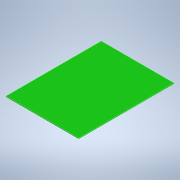
# Autodesk Inventor part: Mock Module PCB
Saved by Autodesk Inventor 2022 (Build 260153000, 153)
## iProperties
Created: 2021-07-19
Part Number: Mock Module PCB
Material: Generic
Document SubType Name: Modeling
Designer: Caleb
Density: 1 g/cm^3
Appearance: Dark Green
Author: Caleb
Autodesk Inventor part; units mm, degrees
(part 1 of 3)
ref_plane "YZ Plane" through (0, 0, 0) normal (1, 0, 0) x (0, 1, 0)
ref_plane "XZ Plane" through (0, 0, 0) normal (0, 1, 0) x (-1, 0, 0)
ref_plane "XY Plane" through (0, 0, 0) normal (0, 0, 1) x (1, 0, 0)
sketch "Sketch1" plane through (0, 0, 0) normal (0, 1, 0) x (-1, 0, 0)
  line L0 (-21.55, 28.25) -> (21.55, 28.25)
  line L1 (21.55, 28.25) -> (21.55, -28.25)
  line L2 (21.55, -28.25) -> (-21.55, -28.25)
  line L3 (-21.55, -28.25) -> (-21.55, 28.25)
  line L4 (-21.55, 28.25) -> (21.55, -28.25) construction
  line L5 (21.55, 28.25) -> (-21.55, -28.25) construction
  point P0 (0, 0)
  dimension "d0" = 43.1
  dimension "d1" = 56.5
  constraints: 12 end point, 2 midpoint, 2 parallel, 1 horizontal, 1 perpendicular
  measures "d0" distance of L0.start L0.end
  measures "d1" distance of L0.end L1.end
extrude "Extrusion1" add sketch "Sketch1" along normal blind 0.5
sketch "Sketch8" plane through (0, 0, 0) normal (0, -1, 0) x (1, 0, 0)
  line L0 (18.3, 26.35) -> (18.2, 26.35)
  line L1 (18.2, 26.35) -> (18.2, 26.05)
  line L2 (18.2, 26.05) -> (18.3, 26.05)
  line L3 (18.3, 26.05) -> (18.3, 26.35)
  line L4 (21.55, 28.25) -> (21.55, -28.25) projected
  line L5 (-21.55, 28.25) -> (21.55, 28.25) projected
  line L6 (18.05, 26.35) -> (17.95, 26.35)
  line L7 (17.95, 26.35) -> (17.95, 26.05)
  line L8 (17.95, 26.05) -> (18.05, 26.05)
  line L9 (18.05, 26.05) -> (18.05, 26.35)
  line L10 (17.8, 26.35) -> (17.7, 26.35)
  line L11 (17.7, 26.35) -> (17.7, 26.05)
  line L12 (17.7, 26.05) -> (17.8, 26.05)
  line L13 (17.8, 26.05) -> (17.8, 26.35)
  line L14 (17.55, 26.35) -> (17.45, 26.35)
  line L15 (17.45, 26.35) -> (17.45, 26.05)
  line L16 (17.45, 26.05) -> (17.55, 26.05)
  line L17 (17.55, 26.05) -> (17.55, 26.35)
  line L18 (17.3, 26.35) -> (17.2, 26.35)
  line L19 (17.2, 26.35) -> (17.2, 26.05)
  line L20 (17.2, 26.05) -> (17.3, 26.05)
  line L21 (17.3, 26.05) -> (17.3, 26.35)
  line L22 (17.05, 26.35) -> (16.95, 26.35)
  line L23 (16.95, 26.35) -> (16.95, 26.05)
  line L24 (16.95, 26.05) -> (17.05, 26.05)
  line L25 (17.05, 26.05) -> (17.05, 26.35)
  line L26 (16.8, 26.35) -> (16.7, 26.35)
  line L27 (16.7, 26.35) -> (16.7, 26.05)
  line L28 (16.7, 26.05) -> (16.8, 26.05)
  line L29 (16.8, 26.05) -> (16.8, 26.35)
  line L30 (16.55, 26.35) -> (16.45, 26.35)
  line L31 (16.45, 26.35) -> (16.45, 26.05)
  line L32 (16.45, 26.05) -> (16.55, 26.05)
  line L33 (16.55, 26.05) -> (16.55, 26.35)
  line L34 (16.3, 26.35) -> (16.2, 26.35)
  line L35 (16.2, 26.35) -> (16.2, 26.05)
  line L36 (16.2, 26.05) -> (16.3, 26.05)
  line L37 (16.3, 26.05) -> (16.3, 26.35)
  line L38 (16.05, 26.35) -> (15.95, 26.35)
  line L39 (15.95, 26.35) -> (15.95, 26.05)
  line L40 (15.95, 26.05) -> (16.05, 26.05)
  line L41 (16.05, 26.05) -> (16.05, 26.35)
  line L42 (15.8, 26.35) -> (15.7, 26.35)
  line L43 (15.7, 26.35) -> (15.7, 26.05)
  line L44 (15.7, 26.05) -> (15.8, 26.05)
  line L45 (15.8, 26.05) -> (15.8, 26.35)
  line L46 (15.55, 26.35) -> (15.45, 26.35)
  line L47 (15.45, 26.35) -> (15.45, 26.05)
  line L48 (15.45, 26.05) -> (15.55, 26.05)
  line L49 (15.55, 26.05) -> (15.55, 26.35)
  line L50 (15.3, 26.35) -> (15.2, 26.35)
  line L51 (15.2, 26.35) -> (15.2, 26.05)
  line L52 (15.2, 26.05) -> (15.3, 26.05)
  line L53 (15.3, 26.05) -> (15.3, 26.35)
  line L54 (15.05, 26.35) -> (14.95, 26.35)
  line L55 (14.95, 26.35) -> (14.95, 26.05)
  line L56 (14.95, 26.05) -> (15.05, 26.05)
  line L57 (15.05, 26.05) -> (15.05, 26.35)
  line L58 (14.8, 26.35) -> (14.7, 26.35)
  line L59 (14.7, 26.35) -> (14.7, 26.05)
  line L60 (14.7, 26.05) -> (14.8, 26.05)
  line L61 (14.8, 26.05) -> (14.8, 26.35)
  line L62 (14.55, 26.35) -> (14.45, 26.35)
  line L63 (14.45, 26.35) -> (14.45, 26.05)
  line L64 (14.45, 26.05) -> (14.55, 26.05)
  line L65 (14.55, 26.05) -> (14.55, 26.35)
  line L66 (14.3, 26.35) -> (14.2, 26.35)
  line L67 (14.2, 26.35) -> (14.2, 26.05)
  line L68 (14.2, 26.05) -> (14.3, 26.05)
  line L69 (14.3, 26.05) -> (14.3, 26.35)
  line L70 (14.05, 26.35) -> (13.95, 26.35)
  line L71 (13.95, 26.35) -> (13.95, 26.05)
  line L72 (13.95, 26.05) -> (14.05, 26.05)
  line L73 (14.05, 26.05) -> (14.05, 26.35)
  line L74 (13.8, 26.35) -> (13.7, 26.35)
  line L75 (13.7, 26.35) -> (13.7, 26.05)
  line L76 (13.7, 26.05) -> (13.8, 26.05)
  line L77 (13.8, 26.05) -> (13.8, 26.35)
  line L78 (13.55, 26.35) -> (13.45, 26.35)
  line L79 (13.45, 26.35) -> (13.45, 26.05)
  line L80 (13.45, 26.05) -> (13.55, 26.05)
  line L81 (13.55, 26.05) -> (13.55, 26.35)
  line L82 (13.3, 26.35) -> (13.2, 26.35)
  line L83 (13.2, 26.35) -> (13.2, 26.05)
  line L84 (13.2, 26.05) -> (13.3, 26.05)
  line L85 (13.3, 26.05) -> (13.3, 26.35)
  line L86 (13.05, 26.35) -> (12.95, 26.35)
  line L87 (12.95, 26.35) -> (12.95, 26.05)
  line L88 (12.95, 26.05) -> (13.05, 26.05)
  line L89 (13.05, 26.05) -> (13.05, 26.35)
  line L90 (12.8, 26.35) -> (12.7, 26.35)
  line L91 (12.7, 26.35) -> (12.7, 26.05)
  line L92 (12.7, 26.05) -> (12.8, 26.05)
  line L93 (12.8, 26.05) -> (12.8, 26.35)
  line L94 (12.55, 26.35) -> (12.45, 26.35)
  line L95 (12.45, 26.35) -> (12.45, 26.05)
  line L96 (12.45, 26.05) -> (12.55, 26.05)
  line L97 (12.55, 26.05) -> (12.55, 26.35)
  line L98 (12.3, 26.35) -> (12.2, 26.35)
  line L99 (12.2, 26.35) -> (12.2, 26.05)
  line L100 (12.2, 26.05) -> (12.3, 26.05)
  line L101 (12.3, 26.05) -> (12.3, 26.35)
  line L102 (12.05, 26.35) -> (11.95, 26.35)
  line L103 (11.95, 26.35) -> (11.95, 26.05)
  line L104 (11.95, 26.05) -> (12.05, 26.05)
  line L105 (12.05, 26.05) -> (12.05, 26.35)
  line L106 (11.8, 26.35) -> (11.7, 26.35)
  line L107 (11.7, 26.35) -> (11.7, 26.05)
  line L108 (11.7, 26.05) -> (11.8, 26.05)
  line L109 (11.8, 26.05) -> (11.8, 26.35)
  line L110 (11.55, 26.35) -> (11.45, 26.35)
  line L111 (11.45, 26.35) -> (11.45, 26.05)
  line L112 (11.45, 26.05) -> (11.55, 26.05)
  line L113 (11.55, 26.05) -> (11.55, 26.35)
  line L114 (11.3, 26.35) -> (11.2, 26.35)
  line L115 (11.2, 26.35) -> (11.2, 26.05)
  line L116 (11.2, 26.05) -> (11.3, 26.05)
  line L117 (11.3, 26.05) -> (11.3, 26.35)
  line L118 (11.05, 26.35) -> (10.95, 26.35)
  line L119 (10.95, 26.35) -> (10.95, 26.05)
  line L120 (10.95, 26.05) -> (11.05, 26.05)
  line L121 (11.05, 26.05) -> (11.05, 26.35)
  line L122 (10.8, 26.35) -> (10.7, 26.35)
  line L123 (10.7, 26.35) -> (10.7, 26.05)
  line L124 (10.7, 26.05) -> (10.8, 26.05)
  line L125 (10.8, 26.05) -> (10.8, 26.35)
  line L126 (10.55, 26.35) -> (10.45, 26.35)
  line L127 (10.45, 26.35) -> (10.45, 26.05)
  line L128 (10.45, 26.05) -> (10.55, 26.05)
  line L129 (10.55, 26.05) -> (10.55, 26.35)
  line L130 (10.3, 26.35) -> (10.2, 26.35)
  line L131 (10.2, 26.35) -> (10.2, 26.05)
  line L132 (10.2, 26.05) -> (10.3, 26.05)
  line L133 (10.3, 26.05) -> (10.3, 26.35)
  line L134 (10.05, 26.35) -> (9.95, 26.35)
  line L135 (9.95, 26.35) -> (9.95, 26.05)
  line L136 (9.95, 26.05) -> (10.05, 26.05)
  line L137 (10.05, 26.05) -> (10.05, 26.35)
  line L138 (9.8, 26.35) -> (9.7, 26.35)
  line L139 (9.7, 26.35) -> (9.7, 26.05)
  line L140 (9.7, 26.05) -> (9.8, 26.05)
  line L141 (9.8, 26.05) -> (9.8, 26.35)
  line L142 (9.55, 26.35) -> (9.45, 26.35)
  line L143 (9.45, 26.35) -> (9.45, 26.05)
  line L144 (9.45, 26.05) -> (9.55, 26.05)
  line L145 (9.55, 26.05) -> (9.55, 26.35)
  line L146 (9.3, 26.35) -> (9.2, 26.35)
  line L147 (9.2, 26.35) -> (9.2, 26.05)
  line L148 (9.2, 26.05) -> (9.3, 26.05)
  line L149 (9.3, 26.05) -> (9.3, 26.35)
  line L150 (9.05, 26.35) -> (8.95, 26.35)
  line L151 (8.95, 26.35) -> (8.95, 26.05)
  line L152 (8.95, 26.05) -> (9.05, 26.05)
  line L153 (9.05, 26.05) -> (9.05, 26.35)
  line L154 (8.8, 26.35) -> (8.7, 26.35)
  line L155 (8.7, 26.35) -> (8.7, 26.05)
  line L156 (8.7, 26.05) -> (8.8, 26.05)
  line L157 (8.8, 26.05) -> (8.8, 26.35)
  line L158 (8.55, 26.35) -> (8.45, 26.35)
  line L159 (8.45, 26.35) -> (8.45, 26.05)
  line L160 (8.45, 26.05) -> (8.55, 26.05)
  line L161 (8.55, 26.05) -> (8.55, 26.35)
  line L162 (8.3, 26.35) -> (8.2, 26.35)
  line L163 (8.2, 26.35) -> (8.2, 26.05)
  line L164 (8.2, 26.05) -> (8.3, 26.05)
  line L165 (8.3, 26.05) -> (8.3, 26.35)
  line L166 (8.05, 26.35) -> (7.95, 26.35)
  line L167 (7.95, 26.35) -> (7.95, 26.05)
  line L168 (7.95, 26.05) -> (8.05, 26.05)
  line L169 (8.05, 26.05) -> (8.05, 26.35)
  line L170 (7.8, 26.35) -> (7.7, 26.35)
  line L171 (7.7, 26.35) -> (7.7, 26.05)
  line L172 (7.7, 26.05) -> (7.8, 26.05)
  line L173 (7.8, 26.05) -> (7.8, 26.35)
  line L174 (7.55, 26.35) -> (7.45, 26.35)
  line L175 (7.45, 26.35) -> (7.45, 26.05)
  line L176 (7.45, 26.05) -> (7.55, 26.05)
  line L177 (7.55, 26.05) -> (7.55, 26.35)
  line L178 (7.3, 26.35) -> (7.2, 26.35)
  line L179 (7.2, 26.35) -> (7.2, 26.05)
  line L180 (7.2, 26.05) -> (7.3, 26.05)
  line L181 (7.3, 26.05) -> (7.3, 26.35)
  line L182 (7.05, 26.35) -> (6.95, 26.35)
  line L183 (6.95, 26.35) -> (6.95, 26.05)
  line L184 (6.95, 26.05) -> (7.05, 26.05)
  line L185 (7.05, 26.05) -> (7.05, 26.35)
  line L186 (6.8, 26.35) -> (6.7, 26.35)
  line L187 (6.7, 26.35) -> (6.7, 26.05)
  line L188 (6.7, 26.05) -> (6.8, 26.05)
  line L189 (6.8, 26.05) -> (6.8, 26.35)
  line L190 (6.55, 26.35) -> (6.45, 26.35)
  line L191 (6.45, 26.35) -> (6.45, 26.05)
  line L192 (6.45, 26.05) -> (6.55, 26.05)
  line L193 (6.55, 26.05) -> (6.55, 26.35)
  line L194 (6.3, 26.35) -> (6.2, 26.35)
  line L195 (6.2, 26.35) -> (6.2, 26.05)
  line L196 (6.2, 26.05) -> (6.3, 26.05)
  line L197 (6.3, 26.05) -> (6.3, 26.35)
  line L198 (6.05, 26.35) -> (5.95, 26.35)
  line L199 (5.95, 26.35) -> (5.95, 26.05)
  line L200 (5.95, 26.05) -> (6.05, 26.05)
  line L201 (6.05, 26.05) -> (6.05, 26.35)
  line L202 (5.8, 26.35) -> (5.7, 26.35)
  line L203 (5.7, 26.35) -> (5.7, 26.05)
  line L204 (5.7, 26.05) -> (5.8, 26.05)
  line L205 (5.8, 26.05) -> (5.8, 26.35)
  line L206 (5.55, 26.35) -> (5.45, 26.35)
  line L207 (5.45, 26.35) -> (5.45, 26.05)
  line L208 (5.45, 26.05) -> (5.55, 26.05)
  line L209 (5.55, 26.05) -> (5.55, 26.35)
  line L210 (5.3, 26.35) -> (5.2, 26.35)
  line L211 (5.2, 26.35) -> (5.2, 26.05)
  line L212 (5.2, 26.05) -> (5.3, 26.05)
  line L213 (5.3, 26.05) -> (5.3, 26.35)
  line L214 (5.05, 26.35) -> (4.95, 26.35)
  line L215 (4.95, 26.35) -> (4.95, 26.05)
  line L216 (4.95, 26.05) -> (5.05, 26.05)
  line L217 (5.05, 26.05) -> (5.05, 26.35)
  line L218 (4.8, 26.35) -> (4.7, 26.35)
  line L219 (4.7, 26.35) -> (4.7, 26.05)
  line L220 (4.7, 26.05) -> (4.8, 26.05)
  line L221 (4.8, 26.05) -> (4.8, 26.35)
  line L222 (4.55, 26.35) -> (4.45, 26.35)
  line L223 (4.45, 26.35) -> (4.45, 26.05)
  line L224 (4.45, 26.05) -> (4.55, 26.05)
  line L225 (4.55, 26.05) -> (4.55, 26.35)
  line L226 (4.3, 26.35) -> (4.2, 26.35)
  line L227 (4.2, 26.35) -> (4.2, 26.05)
  line L228 (4.2, 26.05) -> (4.3, 26.05)
  line L229 (4.3, 26.05) -> (4.3, 26.35)
  line L230 (4.05, 26.35) -> (3.95, 26.35)
  line L231 (3.95, 26.35) -> (3.95, 26.05)
  line L232 (3.95, 26.05) -> (4.05, 26.05)
  line L233 (4.05, 26.05) -> (4.05, 26.35)
  line L234 (3.8, 26.35) -> (3.7, 26.35)
  line L235 (3.7, 26.35) -> (3.7, 26.05)
  line L236 (3.7, 26.05) -> (3.8, 26.05)
  line L237 (3.8, 26.05) -> (3.8, 26.35)
  line L238 (3.55, 26.35) -> (3.45, 26.35)
  line L239 (3.45, 26.35) -> (3.45, 26.05)
  line L240 (3.45, 26.05) -> (3.55, 26.05)
  line L241 (3.55, 26.05) -> (3.55, 26.35)
  line L242 (3.3, 26.35) -> (3.2, 26.35)
  line L243 (3.2, 26.35) -> (3.2, 26.05)
  line L244 (3.2, 26.05) -> (3.3, 26.05)
  line L245 (3.3, 26.05) -> (3.3, 26.35)
  line L246 (3.05, 26.35) -> (2.95, 26.35)
  line L247 (2.95, 26.35) -> (2.95, 26.05)
  line L248 (2.95, 26.05) -> (3.05, 26.05)
  line L249 (3.05, 26.05) -> (3.05, 26.35)
  line L250 (2.8, 26.35) -> (2.7, 26.35)
  line L251 (2.7, 26.35) -> (2.7, 26.05)
  line L252 (2.7, 26.05) -> (2.8, 26.05)
  line L253 (2.8, 26.05) -> (2.8, 26.35)
  line L254 (2.55, 26.35) -> (2.45, 26.35)
  line L255 (2.45, 26.35) -> (2.45, 26.05)
  line L256 (2.45, 26.05) -> (2.55, 26.05)
  line L257 (2.55, 26.05) -> (2.55, 26.35)
  line L258 (2.3, 26.35) -> (2.2, 26.35)
  line L259 (2.2, 26.35) -> (2.2, 26.05)
  line L260 (2.2, 26.05) -> (2.3, 26.05)
  line L261 (2.3, 26.05) -> (2.3, 26.35)
  line L262 (2.05, 26.35) -> (1.95, 26.35)
  line L263 (1.95, 26.35) -> (1.95, 26.05)
  line L264 (1.95, 26.05) -> (2.05, 26.05)
  line L265 (2.05, 26.05) -> (2.05, 26.35)
  line L266 (1.8, 26.35) -> (1.7, 26.35)
  line L267 (1.7, 26.35) -> (1.7, 26.05)
  line L268 (1.7, 26.05) -> (1.8, 26.05)
  line L269 (1.8, 26.05) -> (1.8, 26.35)
  line L270 (1.55, 26.35) -> (1.45, 26.35)
  line L271 (1.45, 26.35) -> (1.45, 26.05)
  line L272 (1.45, 26.05) -> (1.55, 26.05)
  line L273 (1.55, 26.05) -> (1.55, 26.35)
  line L274 (1.3, 26.35) -> (1.2, 26.35)
  line L275 (1.2, 26.35) -> (1.2, 26.05)
  line L276 (1.2, 26.05) -> (1.3, 26.05)
  line L277 (1.3, 26.05) -> (1.3, 26.35)
  line L278 (1.05, 26.35) -> (0.95, 26.35)
  line L279 (0.95, 26.35) -> (0.95, 26.05)
  line L280 (0.95, 26.05) -> (1.05, 26.05)
  line L281 (1.05, 26.05) -> (1.05, 26.35)
  line L282 (0.8, 26.35) -> (0.7, 26.35)
  line L283 (0.7, 26.35) -> (0.7, 26.05)
  line L284 (0.7, 26.05) -> (0.8, 26.05)
  line L285 (0.8, 26.05) -> (0.8, 26.35)
  line L286 (18.175, 25.9738) -> (18.075, 25.9738)
  line L287 (18.075, 25.9738) -> (18.075, 25.6738)
  line L288 (18.075, 25.6738) -> (18.175, 25.6738)
  line L289 (18.175, 25.6738) -> (18.175, 25.9738)
  line L290 (17.825, 25.9738) -> (17.825, 25.6738)
  line L291 (17.925, 25.9738) -> (17.825, 25.9738)
  line L292 (17.825, 25.6738) -> (17.925, 25.6738)
  line L293 (17.925, 25.6738) -> (17.925, 25.9738)
  line L294 (17.575, 25.9738) -> (17.575, 25.6738)
  line L295 (17.675, 25.9738) -> (17.575, 25.9738)
  line L296 (17.575, 25.6738) -> (17.675, 25.6738)
  line L297 (17.675, 25.6738) -> (17.675, 25.9738)
  line L298 (17.325, 25.9738) -> (17.325, 25.6738)
  line L299 (17.425, 25.9738) -> (17.325, 25.9738)
  line L300 (17.325, 25.6738) -> (17.425, 25.6738)
  line L301 (17.425, 25.6738) -> (17.425, 25.9738)
  line L302 (17.075, 25.9738) -> (17.075, 25.6738)
  line L303 (17.175, 25.9738) -> (17.075, 25.9738)
  line L304 (17.075, 25.6738) -> (17.175, 25.6738)
  line L305 (17.175, 25.6738) -> (17.175, 25.9738)
  line L306 (16.825, 25.9738) -> (16.825, 25.6738)
  line L307 (16.925, 25.9738) -> (16.825, 25.9738)
  line L308 (16.825, 25.6738) -> (16.925, 25.6738)
  line L309 (16.925, 25.6738) -> (16.925, 25.9738)
  line L310 (16.575, 25.9738) -> (16.575, 25.6738)
  line L311 (16.675, 25.9738) -> (16.575, 25.9738)
  line L312 (16.575, 25.6738) -> (16.675, 25.6738)
  line L313 (16.675, 25.6738) -> (16.675, 25.9738)
  line L314 (16.325, 25.9738) -> (16.325, 25.6738)
  line L315 (16.425, 25.9738) -> (16.325, 25.9738)
  line L316 (16.325, 25.6738) -> (16.425, 25.6738)
  line L317 (16.425, 25.6738) -> (16.425, 25.9738)
  line L318 (16.075, 25.9738) -> (16.075, 25.6738)
  line L319 (16.175, 25.9738) -> (16.075, 25.9738)
  line L320 (16.075, 25.6738) -> (16.175, 25.6738)
  line L321 (16.175, 25.6738) -> (16.175, 25.9738)
  line L322 (15.825, 25.9738) -> (15.825, 25.6738)
  line L323 (15.925, 25.9738) -> (15.825, 25.9738)
  line L324 (15.825, 25.6738) -> (15.925, 25.6738)
  line L325 (15.925, 25.6738) -> (15.925, 25.9738)
  line L326 (15.575, 25.9738) -> (15.575, 25.6738)
  line L327 (15.675, 25.9738) -> (15.575, 25.9738)
  line L328 (15.575, 25.6738) -> (15.675, 25.6738)
  line L329 (15.675, 25.6738) -> (15.675, 25.9738)
  line L330 (15.325, 25.9738) -> (15.325, 25.6738)
  line L331 (15.425, 25.9738) -> (15.325, 25.9738)
  line L332 (15.325, 25.6738) -> (15.425, 25.6738)
  line L333 (15.425, 25.6738) -> (15.425, 25.9738)
  line L334 (15.075, 25.9738) -> (15.075, 25.6738)
  line L335 (15.175, 25.9738) -> (15.075, 25.9738)
  line L336 (15.075, 25.6738) -> (15.175, 25.6738)
  line L337 (15.175, 25.6738) -> (15.175, 25.9738)
  line L338 (14.825, 25.9738) -> (14.825, 25.6738)
  line L339 (14.925, 25.9738) -> (14.825, 25.9738)
  line L340 (14.825, 25.6738) -> (14.925, 25.6738)
  line L341 (14.925, 25.6738) -> (14.925, 25.9738)
  line L342 (14.575, 25.9738) -> (14.575, 25.6738)
  line L343 (14.675, 25.9738) -> (14.575, 25.9738)
  line L344 (14.575, 25.6738) -> (14.675, 25.6738)
  line L345 (14.675, 25.6738) -> (14.675, 25.9738)
  line L346 (14.325, 25.9738) -> (14.325, 25.6738)
  line L347 (14.425, 25.9738) -> (14.325, 25.9738)
  line L348 (14.325, 25.6738) -> (14.425, 25.6738)
  line L349 (14.425, 25.6738) -> (14.425, 25.9738)
  line L350 (14.075, 25.9738) -> (14.075, 25.6738)
  line L351 (14.175, 25.9738) -> (14.075, 25.9738)
  line L352 (14.075, 25.6738) -> (14.175, 25.6738)
  line L353 (14.175, 25.6738) -> (14.175, 25.9738)
  line L354 (13.825, 25.9738) -> (13.825, 25.6738)
  line L355 (13.925, 25.9738) -> (13.825, 25.9738)
  line L356 (13.825, 25.6738) -> (13.925, 25.6738)
  line L357 (13.925, 25.6738) -> (13.925, 25.9738)
  line L358 (13.575, 25.9738) -> (13.575, 25.6738)
  line L359 (13.675, 25.9738) -> (13.575, 25.9738)
  line L360 (13.575, 25.6738) -> (13.675, 25.6738)
  line L361 (13.675, 25.6738) -> (13.675, 25.9738)
  line L362 (13.325, 25.9738) -> (13.325, 25.6738)
  line L363 (13.425, 25.9738) -> (13.325, 25.9738)
  line L364 (13.325, 25.6738) -> (13.425, 25.6738)
  line L365 (13.425, 25.6738) -> (13.425, 25.9738)
  line L366 (13.075, 25.9738) -> (13.075, 25.6738)
  line L367 (13.175, 25.9738) -> (13.075, 25.9738)
  line L368 (13.075, 25.6738) -> (13.175, 25.6738)
  line L369 (13.175, 25.6738) -> (13.175, 25.9738)
  line L370 (12.825, 25.9738) -> (12.825, 25.6738)
  line L371 (12.925, 25.9738) -> (12.825, 25.9738)
  line L372 (12.825, 25.6738) -> (12.925, 25.6738)
  line L373 (12.925, 25.6738) -> (12.925, 25.9738)
  line L374 (12.575, 25.9738) -> (12.575, 25.6738)
  line L375 (12.675, 25.9738) -> (12.575, 25.9738)
  line L376 (12.575, 25.6738) -> (12.675, 25.6738)
  line L377 (12.675, 25.6738) -> (12.675, 25.9738)
  line L378 (12.325, 25.9738) -> (12.325, 25.6738)
  line L379 (12.425, 25.9738) -> (12.325, 25.9738)
  line L380 (12.325, 25.6738) -> (12.425, 25.6738)
  line L381 (12.425, 25.6738) -> (12.425, 25.9738)
  line L382 (12.075, 25.9738) -> (12.075, 25.6738)
  line L383 (12.175, 25.9738) -> (12.075, 25.9738)
  line L384 (12.075, 25.6738) -> (12.175, 25.6738)
  line L385 (12.175, 25.6738) -> (12.175, 25.9738)
  line L386 (11.825, 25.9738) -> (11.825, 25.6738)
  line L387 (11.925, 25.9738) -> (11.825, 25.9738)
  line L388 (11.825, 25.6738) -> (11.925, 25.6738)
  line L389 (11.925, 25.6738) -> (11.925, 25.9738)
  line L390 (11.575, 25.9738) -> (11.575, 25.6738)
  line L391 (11.675, 25.9738) -> (11.575, 25.9738)
  line L392 (11.575, 25.6738) -> (11.675, 25.6738)
  line L393 (11.675, 25.6738) -> (11.675, 25.9738)
  line L394 (11.325, 25.9738) -> (11.325, 25.6738)
  line L395 (11.425, 25.9738) -> (11.325, 25.9738)
  line L396 (11.325, 25.6738) -> (11.425, 25.6738)
  line L397 (11.425, 25.6738) -> (11.425, 25.9738)
  line L398 (11.075, 25.9738) -> (11.075, 25.6738)
  line L399 (11.175, 25.9738) -> (11.075, 25.9738)
  line L400 (11.075, 25.6738) -> (11.175, 25.6738)
  line L401 (11.175, 25.6738) -> (11.175, 25.9738)
  line L402 (10.825, 25.9738) -> (10.825, 25.6738)
  line L403 (10.925, 25.9738) -> (10.825, 25.9738)
  line L404 (10.825, 25.6738) -> (10.925, 25.6738)
  line L405 (10.925, 25.6738) -> (10.925, 25.9738)
  line L406 (10.575, 25.9738) -> (10.575, 25.6738)
  line L407 (10.675, 25.9738) -> (10.575, 25.9738)
  line L408 (10.575, 25.6738) -> (10.675, 25.6738)
  line L409 (10.675, 25.6738) -> (10.675, 25.9738)
  line L410 (10.325, 25.9738) -> (10.325, 25.6738)
  line L411 (10.425, 25.9738) -> (10.325, 25.9738)
  line L412 (10.325, 25.6738) -> (10.425, 25.6738)
  line L413 (10.425, 25.6738) -> (10.425, 25.9738)
  line L414 (10.075, 25.9738) -> (10.075, 25.6738)
  line L415 (10.175, 25.9738) -> (10.075, 25.9738)
  line L416 (10.075, 25.6738) -> (10.175, 25.6738)
  line L417 (10.175, 25.6738) -> (10.175, 25.9738)
  line L418 (9.825, 25.9738) -> (9.825, 25.6738)
  line L419 (9.925, 25.9738) -> (9.825, 25.9738)
  line L420 (9.825, 25.6738) -> (9.925, 25.6738)
  line L421 (9.925, 25.6738) -> (9.925, 25.9738)
  line L422 (9.575, 25.9738) -> (9.575, 25.6738)
  line L423 (9.675, 25.9738) -> (9.575, 25.9738)
  line L424 (9.575, 25.6738) -> (9.675, 25.6738)
  line L425 (9.675, 25.6738) -> (9.675, 25.9738)
  line L426 (9.325, 25.9738) -> (9.325, 25.6738)
  line L427 (9.425, 25.9738) -> (9.325, 25.9738)
  line L428 (9.325, 25.6738) -> (9.425, 25.6738)
  line L429 (9.425, 25.6738) -> (9.425, 25.9738)
  line L430 (9.075, 25.9738) -> (9.075, 25.6738)
  line L431 (9.175, 25.9738) -> (9.075, 25.9738)
  line L432 (9.075, 25.6738) -> (9.175, 25.6738)
  line L433 (9.175, 25.6738) -> (9.175, 25.9738)
  line L434 (8.825, 25.9738) -> (8.825, 25.6738)
  line L435 (8.925, 25.9738) -> (8.825, 25.9738)
  line L436 (8.825, 25.6738) -> (8.925, 25.6738)
  line L437 (8.925, 25.6738) -> (8.925, 25.9738)
  line L438 (8.575, 25.9738) -> (8.575, 25.6738)
  line L439 (8.675, 25.9738) -> (8.575, 25.9738)
  line L440 (8.575, 25.6738) -> (8.675, 25.6738)
  line L441 (8.675, 25.6738) -> (8.675, 25.9738)
  line L442 (8.325, 25.9738) -> (8.325, 25.6738)
  line L443 (8.425, 25.9738) -> (8.325, 25.9738)
  line L444 (8.325, 25.6738) -> (8.425, 25.6738)
  line L445 (8.425, 25.6738) -> (8.425, 25.9738)
  line L446 (8.075, 25.9738) -> (8.075, 25.6738)
  line L447 (8.175, 25.9738) -> (8.075, 25.9738)
  line L448 (8.075, 25.6738) -> (8.175, 25.6738)
  line L449 (8.175, 25.6738) -> (8.175, 25.9738)
  line L450 (7.825, 25.9738) -> (7.825, 25.6738)
  line L451 (7.925, 25.9738) -> (7.825, 25.9738)
  line L452 (7.825, 25.6738) -> (7.925, 25.6738)
  line L453 (7.925, 25.6738) -> (7.925, 25.9738)
  line L454 (7.575, 25.9738) -> (7.575, 25.6738)
  line L455 (7.675, 25.9738) -> (7.575, 25.9738)
  line L456 (7.575, 25.6738) -> (7.675, 25.6738)
  line L457 (7.675, 25.6738) -> (7.675, 25.9738)
  line L458 (7.325, 25.9738) -> (7.325, 25.6738)
  line L459 (7.425, 25.9738) -> (7.325, 25.9738)
  line L460 (7.325, 25.6738) -> (7.425, 25.6738)
  line L461 (7.425, 25.6738) -> (7.425, 25.9738)
  line L462 (7.075, 25.9738) -> (7.075, 25.6738)
  line L463 (7.175, 25.9738) -> (7.075, 25.9738)
  line L464 (7.075, 25.6738) -> (7.175, 25.6738)
  line L465 (7.175, 25.6738) -> (7.175, 25.9738)
  line L466 (6.825, 25.9738) -> (6.825, 25.6738)
  line L467 (6.925, 25.9738) -> (6.825, 25.9738)
  line L468 (6.825, 25.6738) -> (6.925, 25.6738)
  line L469 (6.925, 25.6738) -> (6.925, 25.9738)
  line L470 (6.575, 25.9738) -> (6.575, 25.6738)
  line L471 (6.675, 25.9738) -> (6.575, 25.9738)
  line L472 (6.575, 25.6738) -> (6.675, 25.6738)
  line L473 (6.675, 25.6738) -> (6.675, 25.9738)
  line L474 (6.325, 25.9738) -> (6.325, 25.6738)
  line L475 (6.425, 25.9738) -> (6.325, 25.9738)
  line L476 (6.325, 25.6738) -> (6.425, 25.6738)
  line L477 (6.425, 25.6738) -> (6.425, 25.9738)
  line L478 (6.075, 25.9738) -> (6.075, 25.6738)
  line L479 (6.175, 25.9738) -> (6.075, 25.9738)
  line L480 (6.075, 25.6738) -> (6.175, 25.6738)
  line L481 (6.175, 25.6738) -> (6.175, 25.9738)
  line L482 (5.825, 25.9738) -> (5.825, 25.6738)
  line L483 (5.925, 25.9738) -> (5.825, 25.9738)
  line L484 (5.825, 25.6738) -> (5.925, 25.6738)
  line L485 (5.925, 25.6738) -> (5.925, 25.9738)
  line L486 (5.575, 25.9738) -> (5.575, 25.6738)
  line L487 (5.675, 25.9738) -> (5.575, 25.9738)
  line L488 (5.575, 25.6738) -> (5.675, 25.6738)
  line L489 (5.675, 25.6738) -> (5.675, 25.9738)
  line L490 (5.325, 25.9738) -> (5.325, 25.6738)
  line L491 (5.425, 25.9738) -> (5.325, 25.9738)
  line L492 (5.325, 25.6738) -> (5.425, 25.6738)
  line L493 (5.425, 25.6738) -> (5.425, 25.9738)
  line L494 (5.075, 25.9738) -> (5.075, 25.6738)
  line L495 (5.175, 25.9738) -> (5.075, 25.9738)
  line L496 (5.075, 25.6738) -> (5.175, 25.6738)
  line L497 (5.175, 25.6738) -> (5.175, 25.9738)
  line L498 (4.825, 25.9738) -> (4.825, 25.6738)
  line L499 (4.925, 25.9738) -> (4.825, 25.9738)
  line L500 (4.825, 25.6738) -> (4.925, 25.6738)
  line L501 (4.925, 25.6738) -> (4.925, 25.9738)
  line L502 (4.575, 25.9738) -> (4.575, 25.6738)
  line L503 (4.675, 25.9738) -> (4.575, 25.9738)
  line L504 (4.575, 25.6738) -> (4.675, 25.6738)
  line L505 (4.675, 25.6738) -> (4.675, 25.9738)
  line L506 (4.325, 25.9738) -> (4.325, 25.6738)
  line L507 (4.425, 25.9738) -> (4.325, 25.9738)
  line L508 (4.325, 25.6738) -> (4.425, 25.6738)
  line L509 (4.425, 25.6738) -> (4.425, 25.9738)
  line L510 (4.075, 25.9738) -> (4.075, 25.6738)
  line L511 (4.175, 25.9738) -> (4.075, 25.9738)
  line L512 (4.075, 25.6738) -> (4.175, 25.6738)
  line L513 (4.175, 25.6738) -> (4.175, 25.9738)
  line L514 (3.825, 25.9738) -> (3.825, 25.6738)
  line L515 (3.925, 25.9738) -> (3.825, 25.9738)
  line L516 (3.825, 25.6738) -> (3.925, 25.6738)
  line L517 (3.925, 25.6738) -> (3.925, 25.9738)
  line L518 (3.575, 25.9738) -> (3.575, 25.6738)
  line L519 (3.675, 25.9738) -> (3.575, 25.9738)
  line L520 (3.575, 25.6738) -> (3.675, 25.6738)
  line L521 (3.675, 25.6738) -> (3.675, 25.9738)
  line L522 (3.325, 25.9738) -> (3.325, 25.6738)
  line L523 (3.425, 25.9738) -> (3.325, 25.9738)
  line L524 (3.325, 25.6738) -> (3.425, 25.6738)
  line L525 (3.425, 25.6738) -> (3.425, 25.9738)
  line L526 (3.075, 25.9738) -> (3.075, 25.6738)
  line L527 (3.175, 25.9738) -> (3.075, 25.9738)
  line L528 (3.075, 25.6738) -> (3.175, 25.6738)
  line L529 (3.175, 25.6738) -> (3.175, 25.9738)
  line L530 (2.825, 25.9738) -> (2.825, 25.6738)
  line L531 (2.925, 25.9738) -> (2.825, 25.9738)
  line L532 (2.825, 25.6738) -> (2.925, 25.6738)
  line L533 (2.925, 25.6738) -> (2.925, 25.9738)
  line L534 (2.575, 25.9738) -> (2.575, 25.6738)
  line L535 (2.675, 25.9738) -> (2.575, 25.9738)
  line L536 (2.575, 25.6738) -> (2.675, 25.6738)
  line L537 (2.675, 25.6738) -> (2.675, 25.9738)
  line L538 (2.325, 25.9738) -> (2.325, 25.6738)
  line L539 (2.425, 25.9738) -> (2.325, 25.9738)
  line L540 (2.325, 25.6738) -> (2.425, 25.6738)
  line L541 (2.425, 25.6738) -> (2.425, 25.9738)
  line L542 (2.075, 25.9738) -> (2.075, 25.6738)
  line L543 (2.175, 25.9738) -> (2.075, 25.9738)
  line L544 (2.075, 25.6738) -> (2.175, 25.6738)
  line L545 (2.175, 25.6738) -> (2.175, 25.9738)
  line L546 (1.825, 25.9738) -> (1.825, 25.6738)
  line L547 (1.925, 25.9738) -> (1.825, 25.9738)
  line L548 (1.825, 25.6738) -> (1.925, 25.6738)
  line L549 (1.925, 25.6738) -> (1.925, 25.9738)
  line L550 (1.575, 25.9738) -> (1.575, 25.6738)
  line L551 (1.675, 25.9738) -> (1.575, 25.9738)
  line L552 (1.575, 25.6738) -> (1.675, 25.6738)
  line L553 (1.675, 25.6738) -> (1.675, 25.9738)
  line L554 (1.325, 25.9738) -> (1.325, 25.6738)
  line L555 (1.425, 25.9738) -> (1.325, 25.9738)
  line L556 (1.325, 25.6738) -> (1.425, 25.6738)
  line L557 (1.425, 25.6738) -> (1.425, 25.9738)
  line L558 (1.075, 25.9738) -> (1.075, 25.6738)
  line L559 (1.175, 25.9738) -> (1.075, 25.9738)
  line L560 (1.075, 25.6738) -> (1.175, 25.6738)
  line L561 (1.175, 25.6738) -> (1.175, 25.9738)
  line L562 (0.825, 25.9738) -> (0.825, 25.6738)
  line L563 (0.925, 25.9738) -> (0.825, 25.9738)
  line L564 (0.825, 25.6738) -> (0.925, 25.6738)
  line L565 (0.925, 25.6738) -> (0.925, 25.9738)
  line L566 (0.575, 25.9738) -> (0.575, 25.6738)
  line L567 (0.675, 25.9738) -> (0.575, 25.9738)
  line L568 (0.575, 25.6738) -> (0.675, 25.6738)
  line L569 (0.675, 25.6738) -> (0.675, 25.9738)
  line L570 (-3.3, 26.35) -> (-3.4, 26.35)
  line L571 (-3.4, 26.35) -> (-3.4, 26.05)
  line L572 (-3.4, 26.05) -> (-3.3, 26.05)
  line L573 (-3.3, 26.05) -> (-3.3, 26.35)
  line L574 (-13.05, 26.35) -> (-13.15, 26.35)
  line L575 (-12.675, 25.9738) -> (-12.775, 25.9738)
  line L576 (-12.925, 25.9738) -> (-13.025, 25.9738)
  line L577 (-12.675, 25.6738) -> (-12.675, 25.9738)
  line L578 (-12.775, 25.6738) -> (-12.675, 25.6738)
  line L579 (-12.775, 25.9738) -> (-12.775, 25.6738)
  line L580 (-12.925, 25.6738) -> (-12.925, 25.9738)
  line L581 (-13.025, 25.6738) -> (-12.925, 25.6738)
  line L582 (-13.025, 25.9738) -> (-13.025, 25.6738)
  line L583 (-13.675, 25.9738) -> (-13.775, 25.9738)
  line L584 (-13.675, 25.6738) -> (-13.675, 25.9738)
  line L585 (-13.775, 25.6738) -> (-13.675, 25.6738)
  line L586 (-13.775, 25.9738) -> (-13.775, 25.6738)
  line L587 (-13.925, 25.9738) -> (-14.025, 25.9738)
  line L588 (-13.925, 25.6738) -> (-13.925, 25.9738)
  line L589 (-14.025, 25.9738) -> (-14.025, 25.6738)
  line L590 (-14.025, 25.6738) -> (-13.925, 25.6738)
  line L591 (-14.675, 25.9738) -> (-14.775, 25.9738)
  line L592 (-14.925, 25.9738) -> (-15.025, 25.9738)
  line L593 (-14.675, 25.6738) -> (-14.675, 25.9738)
  line L594 (-14.775, 25.6738) -> (-14.675, 25.6738)
  line L595 (-14.775, 25.9738) -> (-14.775, 25.6738)
  line L596 (-14.925, 25.6738) -> (-14.925, 25.9738)
  line L597 (-15.025, 25.6738) -> (-14.925, 25.6738)
  line L598 (-15.175, 25.6738) -> (-15.175, 25.9738)
  line L599 (-15.025, 25.9738) -> (-15.025, 25.6738)
  line L600 (-15.675, 25.9738) -> (-15.775, 25.9738)
  line L601 (-15.425, 25.9738) -> (-15.525, 25.9738)
  line L602 (-15.775, 25.9738) -> (-15.775, 25.6738)
  line L603 (-15.775, 25.6738) -> (-15.675, 25.6738)
  line L604 (-15.675, 25.6738) -> (-15.675, 25.9738)
  line L605 (-15.525, 25.9738) -> (-15.525, 25.6738)
  line L606 (-15.175, 25.9738) -> (-15.275, 25.9738)
  line L607 (-15.425, 25.6738) -> (-15.425, 25.9738)
  line L608 (-15.525, 25.6738) -> (-15.425, 25.6738)
  line L609 (-15.275, 25.9738) -> (-15.275, 25.6738)
  line L610 (-15.275, 25.6738) -> (-15.175, 25.6738)
  line L611 (-16.425, 25.9738) -> (-16.525, 25.9738)
  line L612 (-16.675, 25.9738) -> (-16.775, 25.9738)
  line L613 (-16.775, 25.9738) -> (-16.775, 25.6738)
  line L614 (-16.775, 25.6738) -> (-16.675, 25.6738)
  line L615 (-16.525, 25.9738) -> (-16.525, 25.6738)
  line L616 (-16.425, 25.6738) -> (-16.425, 25.9738)
  line L617 (-16.525, 25.6738) -> (-16.425, 25.6738)
  line L618 (-16.675, 25.6738) -> (-16.675, 25.9738)
  line L619 (-17.675, 25.9738) -> (-17.775, 25.9738)
  line L620 (-17.425, 25.9738) -> (-17.525, 25.9738)
  line L621 (-17.425, 25.6738) -> (-17.425, 25.9738)
  line L622 (-17.525, 25.6738) -> (-17.425, 25.6738)
  line L623 (-17.525, 25.9738) -> (-17.525, 25.6738)
  line L624 (-17.675, 25.6738) -> (-17.675, 25.9738)
  line L625 (-17.775, 25.6738) -> (-17.675, 25.6738)
  line L626 (-17.775, 25.9738) -> (-17.775, 25.6738)
  line L627 (-18.425, 25.9738) -> (-18.525, 25.9738)
  line L628 (-18.675, 25.9738) -> (-18.775, 25.9738)
  line L629 (-18.775, 25.6738) -> (-18.675, 25.6738)
  line L630 (-18.775, 25.9738) -> (-18.775, 25.6738)
  line L631 (-18.675, 25.6738) -> (-18.675, 25.9738)
  line L632 (-18.425, 25.6738) -> (-18.425, 25.9738)
  line L633 (-18.525, 25.6738) -> (-18.425, 25.6738)
  line L634 (-18.525, 25.9738) -> (-18.525, 25.6738)
  line L635 (-19.675, 25.9738) -> (-19.775, 25.9738)
  line L636 (-19.675, 25.6738) -> (-19.675, 25.9738)
  line L637 (-19.775, 25.6738) -> (-19.675, 25.6738)
  line L638 (-19.925, 25.9738) -> (-20.025, 25.9738)
  line L639 (-19.775, 25.9738) -> (-19.775, 25.6738)
  line L640 (-19.925, 25.6738) -> (-19.925, 25.9738)
  line L641 (-20.025, 25.9738) -> (-20.025, 25.6738)
  line L642 (-20.025, 25.6738) -> (-19.925, 25.6738)
  line L643 (-20.675, 25.9738) -> (-20.775, 25.9738)
  line L644 (-20.675, 25.6738) -> (-20.675, 25.9738)
  line L645 (-20.775, 25.6738) -> (-20.675, 25.6738)
  line L646 (-20.925, 25.9738) -> (-21.025, 25.9738)
  line L647 (-20.925, 25.6738) -> (-20.925, 25.9738)
  line L648 (-21.025, 25.9738) -> (-21.025, 25.6738)
  line L649 (-21.025, 25.6738) -> (-20.925, 25.6738)
  line L650 (-20.775, 25.9738) -> (-20.775, 25.6738)
  line L651 (-12.175, 25.6738) -> (-12.175, 25.9738)
  line L652 (-12.175, 25.9738) -> (-12.275, 25.9738)
  line L653 (-12.275, 25.6738) -> (-12.175, 25.6738)
  line L654 (-12.275, 25.9738) -> (-12.275, 25.6738)
  line L655 (-12.425, 25.6738) -> (-12.425, 25.9738)
  line L656 (-12.525, 25.9738) -> (-12.525, 25.6738)
  line L657 (-12.525, 25.6738) -> (-12.425, 25.6738)
  line L658 (-12.425, 25.9738) -> (-12.525, 25.9738)
  line L659 (-12.3, 26.35) -> (-12.4, 26.35)
  line L660 (-12.4, 26.35) -> (-12.4, 26.05)
  line L661 (-12.4, 26.05) -> (-12.3, 26.05)
  line L662 (-12.9, 26.05) -> (-12.8, 26.05)
  line L663 (-12.65, 26.05) -> (-12.55, 26.05)
  line L664 (-12.9, 26.35) -> (-12.9, 26.05)
  line L665 (-12.8, 26.05) -> (-12.8, 26.35)
  line L666 (-12.65, 26.35) -> (-12.65, 26.05)
  line L667 (-12.55, 26.05) -> (-12.55, 26.35)
  line L668 (-12.3, 26.05) -> (-12.3, 26.35)
  line L669 (-12.55, 26.35) -> (-12.65, 26.35)
  line L670 (-12.8, 26.35) -> (-12.9, 26.35)
  line L671 (-13.175, 25.6738) -> (-13.175, 25.9738)
  line L672 (-13.175, 25.9738) -> (-13.275, 25.9738)
  line L673 (-13.275, 25.6738) -> (-13.175, 25.6738)
  line L674 (-13.275, 25.9738) -> (-13.275, 25.6738)
  line L675 (-13.425, 25.6738) -> (-13.425, 25.9738)
  line L676 (-13.525, 25.9738) -> (-13.525, 25.6738)
  line L677 (-13.525, 25.6738) -> (-13.425, 25.6738)
  line L678 (-13.425, 25.9738) -> (-13.525, 25.9738)
  line L679 (-13.3, 26.35) -> (-13.4, 26.35)
  line L680 (-13.55, 26.35) -> (-13.65, 26.35)
  line L681 (-13.15, 26.05) -> (-13.05, 26.05)
  line L682 (-13.05, 26.05) -> (-13.05, 26.35)
  line L683 (-13.15, 26.35) -> (-13.15, 26.05)
  line L684 (-13.4, 26.05) -> (-13.3, 26.05)
  line L685 (-13.3, 26.05) -> (-13.3, 26.35)
  line L686 (-13.4, 26.35) -> (-13.4, 26.05)
  line L687 (-13.65, 26.05) -> (-13.55, 26.05)
  line L688 (-13.55, 26.05) -> (-13.55, 26.35)
  line L689 (-13.65, 26.35) -> (-13.65, 26.05)
  line L690 (-13.9, 26.05) -> (-13.8, 26.05)
  line L691 (-13.8, 26.05) -> (-13.8, 26.35)
  line L692 (-13.9, 26.35) -> (-13.9, 26.05)
  line L693 (-13.8, 26.35) -> (-13.9, 26.35)
  line L694 (-14.05, 26.35) -> (-14.15, 26.35)
  line L695 (-14.15, 26.35) -> (-14.15, 26.05)
  line L696 (-14.15, 26.05) -> (-14.05, 26.05)
  line L697 (-14.05, 26.05) -> (-14.05, 26.35)
  line L698 (-14.3, 26.35) -> (-14.4, 26.35)
  line L699 (-14.4, 26.35) -> (-14.4, 26.05)
  line L700 (-14.4, 26.05) -> (-14.3, 26.05)
  line L701 (-14.3, 26.05) -> (-14.3, 26.35)
  line L702 (-14.9, 26.05) -> (-14.8, 26.05)
  line L703 (-14.65, 26.05) -> (-14.55, 26.05)
  line L704 (-14.8, 26.35) -> (-14.9, 26.35)
  line L705 (-14.8, 26.05) -> (-14.8, 26.35)
  line L706 (-14.65, 26.35) -> (-14.65, 26.05)
  line L707 (-14.55, 26.35) -> (-14.65, 26.35)
  line L708 (-14.55, 26.05) -> (-14.55, 26.35)
  line L709 (-14.9, 26.35) -> (-14.9, 26.05)
  line L710 (-15.05, 26.35) -> (-15.15, 26.35)
  line L711 (-15.15, 26.35) -> (-15.15, 26.05)
  line L712 (-15.15, 26.05) -> (-15.05, 26.05)
  line L713 (-15.05, 26.05) -> (-15.05, 26.35)
  line L714 (-15.3, 26.35) -> (-15.4, 26.35)
  line L715 (-15.4, 26.35) -> (-15.4, 26.05)
  line L716 (-15.4, 26.05) -> (-15.3, 26.05)
  line L717 (-15.3, 26.05) -> (-15.3, 26.35)
  line L718 (-15.65, 26.05) -> (-15.55, 26.05)
  line L719 (-15.55, 26.35) -> (-15.65, 26.35)
  line L720 (-15.55, 26.05) -> (-15.55, 26.35)
  line L721 (-15.65, 26.35) -> (-15.65, 26.05)
  line L722 (-15.8, 26.05) -> (-15.8, 26.35)
  line L723 (-15.8, 26.35) -> (-15.9, 26.35)
  line L724 (-15.9, 26.35) -> (-15.9, 26.05)
  line L725 (-15.9, 26.05) -> (-15.8, 26.05)
  line L726 (-16.025, 25.9738) -> (-16.025, 25.6738)
  line L727 (-15.925, 25.9738) -> (-16.025, 25.9738)
  line L728 (-16.025, 25.6738) -> (-15.925, 25.6738)
  line L729 (-16.175, 25.6738) -> (-16.175, 25.9738)
  line L730 (-16.275, 25.9738) -> (-16.275, 25.6738)
  line L731 (-16.275, 25.6738) -> (-16.175, 25.6738)
  line L732 (-16.175, 25.9738) -> (-16.275, 25.9738)
  line L733 (-15.925, 25.6738) -> (-15.925, 25.9738)
  line L734 (-16.05, 26.35) -> (-16.15, 26.35)
  line L735 (-16.15, 26.35) -> (-16.15, 26.05)
  line L736 (-16.15, 26.05) -> (-16.05, 26.05)
  line L737 (-16.05, 26.05) -> (-16.05, 26.35)
  line L738 (-16.3, 26.35) -> (-16.4, 26.35)
  line L739 (-16.4, 26.35) -> (-16.4, 26.05)
  line L740 (-16.4, 26.05) -> (-16.3, 26.05)
  line L741 (-16.65, 26.05) -> (-16.55, 26.05)
  line L742 (-16.9, 26.05) -> (-16.8, 26.05)
  line L743 (-16.3, 26.05) -> (-16.3, 26.35)
  line L744 (-16.55, 26.35) -> (-16.65, 26.35)
  line L745 (-16.55, 26.05) -> (-16.55, 26.35)
  line L746 (-16.65, 26.35) -> (-16.65, 26.05)
  line L747 (-16.8, 26.05) -> (-16.8, 26.35)
  line L748 (-16.9, 26.35) -> (-16.9, 26.05)
  line L749 (-16.8, 26.35) -> (-16.9, 26.35)
  line L750 (-16.925, 25.6738) -> (-16.925, 25.9738)
  line L751 (-17.025, 25.9738) -> (-17.025, 25.6738)
  line L752 (-16.925, 25.9738) -> (-17.025, 25.9738)
  line L753 (-17.025, 25.6738) -> (-16.925, 25.6738)
  line L754 (-17.175, 25.6738) -> (-17.175, 25.9738)
  line L755 (-17.275, 25.9738) -> (-17.275, 25.6738)
  line L756 (-17.175, 25.9738) -> (-17.275, 25.9738)
  line L757 (-17.275, 25.6738) -> (-17.175, 25.6738)
  line L758 (-17.05, 26.35) -> (-17.15, 26.35)
  line L759 (-17.15, 26.35) -> (-17.15, 26.05)
  line L760 (-17.15, 26.05) -> (-17.05, 26.05)
  line L761 (-17.05, 26.05) -> (-17.05, 26.35)
  line L762 (-17.3, 26.35) -> (-17.4, 26.35)
  line L763 (-17.4, 26.35) -> (-17.4, 26.05)
  line L764 (-17.4, 26.05) -> (-17.3, 26.05)
  line L765 (-17.65, 26.05) -> (-17.55, 26.05)
  line L766 (-17.9, 26.05) -> (-17.8, 26.05)
  line L767 (-17.8, 26.35) -> (-17.9, 26.35)
  line L768 (-17.9, 26.35) -> (-17.9, 26.05)
  line L769 (-17.8, 26.05) -> (-17.8, 26.35)
  line L770 (-17.65, 26.35) -> (-17.65, 26.05)
  line L771 (-17.55, 26.35) -> (-17.65, 26.35)
  line L772 (-17.3, 26.05) -> (-17.3, 26.35)
  line L773 (-17.55, 26.05) -> (-17.55, 26.35)
  line L774 (-17.925, 25.6738) -> (-17.925, 25.9738)
  line L775 (-18.025, 25.9738) -> (-18.025, 25.6738)
  line L776 (-17.925, 25.9738) -> (-18.025, 25.9738)
  line L777 (-18.025, 25.6738) -> (-17.925, 25.6738)
  line L778 (-18.175, 25.6738) -> (-18.175, 25.9738)
  line L779 (-18.275, 25.9738) -> (-18.275, 25.6738)
  line L780 (-18.275, 25.6738) -> (-18.175, 25.6738)
  line L781 (-18.175, 25.9738) -> (-18.275, 25.9738)
  line L782 (-18.05, 26.35) -> (-18.15, 26.35)
  line L783 (-18.15, 26.35) -> (-18.15, 26.05)
  line L784 (-18.15, 26.05) -> (-18.05, 26.05)
  line L785 (-18.05, 26.05) -> (-18.05, 26.35)
  line L786 (-18.3, 26.35) -> (-18.4, 26.35)
  line L787 (-18.4, 26.35) -> (-18.4, 26.05)
  line L788 (-18.4, 26.05) -> (-18.3, 26.05)
  line L789 (-18.9, 26.05) -> (-18.8, 26.05)
  line L790 (-18.3, 26.05) -> (-18.3, 26.35)
  line L791 (-18.55, 26.05) -> (-18.55, 26.35)
  line L792 (-18.55, 26.35) -> (-18.65, 26.35)
  line L793 (-18.65, 26.35) -> (-18.65, 26.05)
  line L794 (-18.8, 26.05) -> (-18.8, 26.35)
  line L795 (-18.8, 26.35) -> (-18.9, 26.35)
  line L796 (-18.9, 26.35) -> (-18.9, 26.05)
  line L797 (-18.65, 26.05) -> (-18.55, 26.05)
  line L798 (-18.925, 25.6738) -> (-18.925, 25.9738)
  line L799 (-18.925, 25.9738) -> (-19.025, 25.9738)
  line L800 (-19.025, 25.6738) -> (-18.925, 25.6738)
  line L801 (-19.025, 25.9738) -> (-19.025, 25.6738)
  line L802 (-19.175, 25.6738) -> (-19.175, 25.9738)
  line L803 (-19.175, 25.9738) -> (-19.275, 25.9738)
  line L804 (-19.275, 25.6738) -> (-19.175, 25.6738)
  line L805 (-19.275, 25.9738) -> (-19.275, 25.6738)
  line L806 (-19.425, 25.6738) -> (-19.425, 25.9738)
  line L807 (-19.525, 25.9738) -> (-19.525, 25.6738)
  line L808 (-19.425, 25.9738) -> (-19.525, 25.9738)
  line L809 (-19.525, 25.6738) -> (-19.425, 25.6738)
  line L810 (-19.05, 26.35) -> (-19.15, 26.35)
  line L811 (-19.15, 26.35) -> (-19.15, 26.05)
  line L812 (-19.15, 26.05) -> (-19.05, 26.05)
  line L813 (-19.05, 26.05) -> (-19.05, 26.35)
  line L814 (-19.3, 26.35) -> (-19.4, 26.35)
  line L815 (-19.4, 26.35) -> (-19.4, 26.05)
  line L816 (-19.4, 26.05) -> (-19.3, 26.05)
  line L817 (-19.9, 26.05) -> (-19.8, 26.05)
  line L818 (-19.65, 26.05) -> (-19.55, 26.05)
  line L819 (-19.8, 26.35) -> (-19.9, 26.35)
  line L820 (-19.9, 26.35) -> (-19.9, 26.05)
  line L821 (-19.8, 26.05) -> (-19.8, 26.35)
  line L822 (-19.55, 26.35) -> (-19.65, 26.35)
  line L823 (-19.55, 26.05) -> (-19.55, 26.35)
  line L824 (-19.3, 26.05) -> (-19.3, 26.35)
  line L825 (-19.65, 26.35) -> (-19.65, 26.05)
  line L826 (-20.175, 25.6738) -> (-20.175, 25.9738)
  line L827 (-20.275, 25.6738) -> (-20.175, 25.6738)
  line L828 (-20.175, 25.9738) -> (-20.275, 25.9738)
  line L829 (-20.275, 25.9738) -> (-20.275, 25.6738)
  line L830 (-20.425, 25.6738) -> (-20.425, 25.9738)
  line L831 (-20.525, 25.9738) -> (-20.525, 25.6738)
  line L832 (-20.425, 25.9738) -> (-20.525, 25.9738)
  line L833 (-20.525, 25.6738) -> (-20.425, 25.6738)
  line L834 (-20.05, 26.35) -> (-20.15, 26.35)
  line L835 (-20.15, 26.35) -> (-20.15, 26.05)
  line L836 (-20.15, 26.05) -> (-20.05, 26.05)
  line L837 (-20.05, 26.05) -> (-20.05, 26.35)
  line L838 (-20.3, 26.35) -> (-20.4, 26.35)
  line L839 (-20.4, 26.35) -> (-20.4, 26.05)
  line L840 (-20.4, 26.05) -> (-20.3, 26.05)
  line L841 (-20.9, 26.05) -> (-20.8, 26.05)
  line L842 (-20.65, 26.05) -> (-20.55, 26.05)
  line L843 (-20.8, 26.35) -> (-20.9, 26.35)
  line L844 (-20.9, 26.35) -> (-20.9, 26.05)
  line L845 (-20.8, 26.05) -> (-20.8, 26.35)
  line L846 (-20.65, 26.35) -> (-20.65, 26.05)
  line L847 (-20.55, 26.05) -> (-20.55, 26.35)
  line L848 (-20.3, 26.05) -> (-20.3, 26.35)
  line L849 (-20.55, 26.35) -> (-20.65, 26.35)
  line L850 (-14.175, 25.6738) -> (-14.175, 25.9738)
  line L851 (-14.275, 25.6738) -> (-14.175, 25.6738)
  line L852 (-14.175, 25.9738) -> (-14.275, 25.9738)
  line L853 (-14.275, 25.9738) -> (-14.275, 25.6738)
  line L854 (-14.425, 25.6738) -> (-14.425, 25.9738)
  line L855 (-14.525, 25.9738) -> (-14.525, 25.6738)
  line L856 (-14.425, 25.9738) -> (-14.525, 25.9738)
  line L857 (-14.525, 25.6738) -> (-14.425, 25.6738)
  line L858 (-4.15, 26.35) -> (-4.15, 26.05)
  line L859 (-4.05, 26.35) -> (-4.15, 26.35)
  line L860 (-4.15, 26.05) -> (-4.05, 26.05)
  line L861 (-4.05, 26.05) -> (-4.05, 26.35)
  line L862 (-3.8, 26.35) -> (-3.9, 26.35)
  line L863 (-3.9, 26.05) -> (-3.8, 26.05)
  line L864 (-3.8, 26.05) -> (-3.8, 26.35)
  line L865 (-3.9, 26.35) -> (-3.9, 26.05)
  line L866 (-4.4, 26.05) -> (-4.3, 26.05)
  line L867 (-4.3, 26.35) -> (-4.4, 26.35)
  line L868 (-4.4, 26.35) -> (-4.4, 26.05)
  line L869 (-4.55, 26.05) -> (-4.55, 26.35)
  line L870 (-4.65, 26.05) -> (-4.55, 26.05)
  line L871 (-4.55, 26.35) -> (-4.65, 26.35)
  line L872 (-4.65, 26.35) -> (-4.65, 26.05)
  line L873 (-4.3, 26.05) -> (-4.3, 26.35)
  line L874 (-4.8, 26.35) -> (-4.9, 26.35)
  line L875 (-4.9, 26.35) -> (-4.9, 26.05)
  line L876 (-4.9, 26.05) -> (-4.8, 26.05)
  line L877 (-4.8, 26.05) -> (-4.8, 26.35)
  line L878 (-5.05, 26.35) -> (-5.15, 26.35)
  line L879 (-5.15, 26.35) -> (-5.15, 26.05)
  line L880 (-5.15, 26.05) -> (-5.05, 26.05)
  line L881 (-5.4, 26.05) -> (-5.3, 26.05)
  line L882 (-5.65, 26.05) -> (-5.55, 26.05)
  line L883 (-5.05, 26.05) -> (-5.05, 26.35)
  line L884 (-5.3, 26.05) -> (-5.3, 26.35)
  line L885 (-5.3, 26.35) -> (-5.4, 26.35)
  line L886 (-5.4, 26.35) -> (-5.4, 26.05)
  line L887 (-5.55, 26.05) -> (-5.55, 26.35)
  line L888 (-5.65, 26.35) -> (-5.65, 26.05)
  line L889 (-5.55, 26.35) -> (-5.65, 26.35)
  line L890 (-5.8, 26.35) -> (-5.9, 26.35)
  line L891 (-5.9, 26.35) -> (-5.9, 26.05)
  line L892 (-5.9, 26.05) -> (-5.8, 26.05)
  line L893 (-5.8, 26.05) -> (-5.8, 26.35)
  line L894 (-6.05, 26.35) -> (-6.15, 26.35)
  line L895 (-6.15, 26.35) -> (-6.15, 26.05)
  line L896 (-6.15, 26.05) -> (-6.05, 26.05)
  line L897 (-6.05, 26.05) -> (-6.05, 26.35)
  line L898 (-6.65, 26.05) -> (-6.55, 26.05)
  line L899 (-6.4, 26.05) -> (-6.3, 26.05)
  line L900 (-6.55, 26.35) -> (-6.65, 26.35)
  line L901 (-6.65, 26.35) -> (-6.65, 26.05)
  line L902 (-6.55, 26.05) -> (-6.55, 26.35)
  line L903 (-6.4, 26.35) -> (-6.4, 26.05)
  line L904 (-6.3, 26.35) -> (-6.4, 26.35)
  line L905 (-6.3, 26.05) -> (-6.3, 26.35)
  line L906 (-6.8, 26.35) -> (-6.9, 26.35)
  line L907 (-6.9, 26.35) -> (-6.9, 26.05)
  line L908 (-6.9, 26.05) -> (-6.8, 26.05)
  line L909 (-6.8, 26.05) -> (-6.8, 26.35)
  line L910 (-7.05, 26.35) -> (-7.15, 26.35)
  line L911 (-7.15, 26.35) -> (-7.15, 26.05)
  line L912 (-7.15, 26.05) -> (-7.05, 26.05)
  line L913 (-7.05, 26.05) -> (-7.05, 26.35)
  line L914 (-7.3, 26.35) -> (-7.4, 26.35)
  line L915 (-7.3, 26.05) -> (-7.3, 26.35)
  line L916 (-7.65, 26.05) -> (-7.55, 26.05)
  line L917 (-7.4, 26.35) -> (-7.4, 26.05)
  line L918 (-7.55, 26.05) -> (-7.55, 26.35)
  line L919 (-7.55, 26.35) -> (-7.65, 26.35)
  line L920 (-7.65, 26.35) -> (-7.65, 26.05)
  line L921 (-7.4, 26.05) -> (-7.3, 26.05)
  line L922 (-7.8, 26.35) -> (-7.9, 26.35)
  line L923 (-7.9, 26.35) -> (-7.9, 26.05)
  line L924 (-7.9, 26.05) -> (-7.8, 26.05)
  line L925 (-7.8, 26.05) -> (-7.8, 26.35)
  line L926 (-8.05, 26.35) -> (-8.15, 26.35)
  line L927 (-8.15, 26.35) -> (-8.15, 26.05)
  line L928 (-8.15, 26.05) -> (-8.05, 26.05)
  line L929 (-8.4, 26.05) -> (-8.3, 26.05)
  line L930 (-8.65, 26.05) -> (-8.55, 26.05)
  line L931 (-8.55, 26.35) -> (-8.65, 26.35)
  line L932 (-8.65, 26.35) -> (-8.65, 26.05)
  line L933 (-8.55, 26.05) -> (-8.55, 26.35)
  line L934 (-8.3, 26.35) -> (-8.4, 26.35)
  line L935 (-8.4, 26.35) -> (-8.4, 26.05)
  line L936 (-8.3, 26.05) -> (-8.3, 26.35)
  line L937 (-8.05, 26.05) -> (-8.05, 26.35)
  line L938 (-8.8, 26.35) -> (-8.9, 26.35)
  line L939 (-8.9, 26.35) -> (-8.9, 26.05)
  line L940 (-8.9, 26.05) -> (-8.8, 26.05)
  line L941 (-8.8, 26.05) -> (-8.8, 26.35)
  line L942 (-9.05, 26.35) -> (-9.15, 26.35)
  line L943 (-9.15, 26.35) -> (-9.15, 26.05)
  line L944 (-9.15, 26.05) -> (-9.05, 26.05)
  line L945 (-9.05, 26.05) -> (-9.05, 26.35)
  line L946 (-9.3, 26.35) -> (-9.4, 26.35)
  line L947 (-9.4, 26.35) -> (-9.4, 26.05)
  line L948 (-9.4, 26.05) -> (-9.3, 26.05)
  line L949 (-9.3, 26.05) -> (-9.3, 26.35)
  line L950 (-9.55, 26.35) -> (-9.65, 26.35)
  line L951 (-9.65, 26.35) -> (-9.65, 26.05)
  line L952 (-9.65, 26.05) -> (-9.55, 26.05)
  line L953 (-9.55, 26.05) -> (-9.55, 26.35)
  line L954 (-10.675, 25.9738) -> (-10.775, 25.9738)
  line L955 (-11.025, 25.9738) -> (-11.025, 25.6738)
  line L956 (-10.925, 25.6738) -> (-10.925, 25.9738)
  line L957 (-11.025, 25.6738) -> (-10.925, 25.6738)
  line L958 (-10.775, 25.9738) -> (-10.775, 25.6738)
  line L959 (-10.675, 25.6738) -> (-10.675, 25.9738)
  line L960 (-10.775, 25.6738) -> (-10.675, 25.6738)
  line L961 (-10.925, 25.9738) -> (-11.025, 25.9738)
  line L962 (-11.675, 25.9738) -> (-11.775, 25.9738)
  line L963 (-11.925, 25.9738) -> (-12.025, 25.9738)
  line L964 (-12.025, 25.9738) -> (-12.025, 25.6738)
  line L965 (-11.925, 25.6738) -> (-11.925, 25.9738)
  line L966 (-12.025, 25.6738) -> (-11.925, 25.6738)
  line L967 (-11.775, 25.9738) -> (-11.775, 25.6738)
  line L968 (-11.675, 25.6738) -> (-11.675, 25.9738)
  line L969 (-11.775, 25.6738) -> (-11.675, 25.6738)
  line L970 (-11.3, 26.35) -> (-11.4, 26.35)
  line L971 (-11.4, 26.35) -> (-11.4, 26.05)
  line L972 (-11.4, 26.05) -> (-11.3, 26.05)
  line L973 (-11.3, 26.05) -> (-11.3, 26.35)
  line L974 (-11.55, 26.35) -> (-11.65, 26.35)
  line L975 (-11.65, 26.35) -> (-11.65, 26.05)
  line L976 (-11.65, 26.05) -> (-11.55, 26.05)
  line L977 (-11.9, 26.05) -> (-11.8, 26.05)
  line L978 (-12.15, 26.05) -> (-12.05, 26.05)
  line L979 (-11.55, 26.05) -> (-11.55, 26.35)
  line L980 (-11.8, 26.35) -> (-11.9, 26.35)
  line L981 (-11.8, 26.05) -> (-11.8, 26.35)
  line L982 (-11.9, 26.35) -> (-11.9, 26.05)
  line L983 (-12.05, 26.05) -> (-12.05, 26.35)
  line L984 (-12.05, 26.35) -> (-12.15, 26.35)
  line L985 (-12.15, 26.35) -> (-12.15, 26.05)
  line L986 (-11.175, 25.6738) -> (-11.175, 25.9738)
  line L987 (-11.275, 25.6738) -> (-11.175, 25.6738)
  line L988 (-11.175, 25.9738) -> (-11.275, 25.9738)
  line L989 (-11.275, 25.9738) -> (-11.275, 25.6738)
  line L990 (-11.525, 25.9738) -> (-11.525, 25.6738)
  line L991 (-11.425, 25.9738) -> (-11.525, 25.9738)
  line L992 (-11.525, 25.6738) -> (-11.425, 25.6738)
  line L993 (-11.425, 25.6738) -> (-11.425, 25.9738)
  line L994 (-10.3, 26.35) -> (-10.4, 26.35)
  line L995 (-10.4, 26.35) -> (-10.4, 26.05)
  line L996 (-10.4, 26.05) -> (-10.3, 26.05)
  line L997 (-10.3, 26.05) -> (-10.3, 26.35)
  line L998 (-10.55, 26.35) -> (-10.65, 26.35)
  line L999 (-10.65, 26.35) -> (-10.65, 26.05)
  line L1000 (-10.65, 26.05) -> (-10.55, 26.05)
  line L1001 (-10.9, 26.05) -> (-10.8, 26.05)
  line L1002 (-10.55, 26.05) -> (-10.55, 26.35)
  line L1003 (-10.8, 26.35) -> (-10.9, 26.35)
  line L1004 (-10.8, 26.05) -> (-10.8, 26.35)
  line L1005 (-10.9, 26.35) -> (-10.9, 26.05)
  line L1006 (-11.05, 26.05) -> (-11.05, 26.35)
  line L1007 (-11.05, 26.35) -> (-11.15, 26.35)
  line L1008 (-11.15, 26.35) -> (-11.15, 26.05)
  line L1009 (-11.15, 26.05) -> (-11.05, 26.05)
  line L1010 (-10.175, 25.6738) -> (-10.175, 25.9738)
  line L1011 (-10.175, 25.9738) -> (-10.275, 25.9738)
  line L1012 (-10.275, 25.6738) -> (-10.175, 25.6738)
  line L1013 (-10.425, 25.6738) -> (-10.425, 25.9738)
  line L1014 (-10.525, 25.9738) -> (-10.525, 25.6738)
  line L1015 (-10.425, 25.9738) -> (-10.525, 25.9738)
  line L1016 (-10.525, 25.6738) -> (-10.425, 25.6738)
  line L1017 (-10.275, 25.9738) -> (-10.275, 25.6738)
  line L1018 (-9.8, 26.05) -> (-9.8, 26.35)
  line L1019 (-9.675, 25.9738) -> (-9.775, 25.9738)
  line L1020 (-9.9, 26.05) -> (-9.8, 26.05)
  line L1021 (-9.8, 26.35) -> (-9.9, 26.35)
  line L1022 (-9.9, 26.35) -> (-9.9, 26.05)
  line L1023 (-9.925, 25.9738) -> (-10.025, 25.9738)
  line L1024 (-9.675, 25.6738) -> (-9.675, 25.9738)
  line L1025 (-9.775, 25.6738) -> (-9.675, 25.6738)
  line L1026 (-9.775, 25.9738) -> (-9.775, 25.6738)
  line L1027 (-9.925, 25.6738) -> (-9.925, 25.9738)
  line L1028 (-10.025, 25.6738) -> (-9.925, 25.6738)
  line L1029 (-10.025, 25.9738) -> (-10.025, 25.6738)
  line L1030 (-10.15, 26.05) -> (-10.05, 26.05)